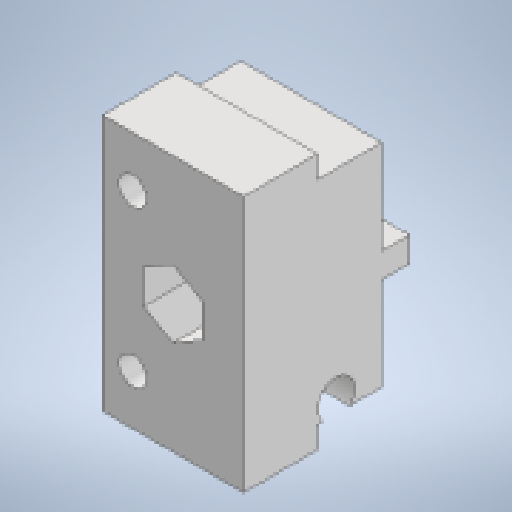
# Autodesk Inventor part: pokrywa silników
Saved by Autodesk Inventor 2023 (Build 270158000, 158)
## iProperties
Created: 2022-12-13
Part Number: pokrywa silników
Material: Generic
Document SubType Name: Modeling
Designer: komputer
Density: 1 g/cm^3
Appearance: Default
Author: komputer
Autodesk Inventor part; units mm, degrees
ref_plane "YZ Plane" through (0, 0, 0) normal (1, 0, 0) x (0, 1, 0)
ref_plane "XZ Plane" through (0, 0, 0) normal (0, 1, 0) x (-1, 0, 0)
ref_plane "XY Plane" through (0, 0, 0) normal (0, 0, 1) x (1, 0, 0)
sketch "Sketch1" plane through (0, 0, 0) normal (0, 0, 1) x (1, 0, 0)
  line L0 (-23.5108, -23.5) -> (0, -23.5) projected
  line L1 (0, -10) -> (0, -23.5) projected
  line L2 (0, -10) -> (-23, -10) projected
  line L3 (-23, 0) -> (-23, -10) projected
  line L4 (-23, 0) -> (7.65, 0) projected
  line L5 (7.65, 3) -> (-23, 3) projected
  line L6 (-23, 13) -> (-23, 3) projected
  line L7 (-23, 13) -> (0, 13) projected
  line L8 (0, 26.5) -> (0, 13) projected
  line L9 (-23.5108, 26.5) -> (0, 26.5) projected
  line L10 (0, 3.8) -> (14.8, 3.8) projected
  line L11 (0, 12.2) -> (14.8, 12.2) projected
  line L12 (14.8, -0.8) -> (0, -0.8) projected
  line L13 (14.8, -9.2) -> (0, -9.2) projected
  line L14 (0, 3.8) -> (0, -0.8)
  circle A0 centre (0, 1.5) radius 3.0601
  line L15 (0, -0.8) -> (3.8745, -4.6745)
  line L16 (0, -0.8) -> (5.4793, -0.8) construction
  line L17 (0, 3.8) -> (3.8745, 7.6745)
  line L18 (0, 3.8) -> (5.4793, 3.8) construction
  line L19 (0.6829, -1.4829) -> (11.7635, -1.4829)
  line L20 (11.7635, -1.4829) -> (11.7635, -8.6829)
  line L21 (11.7635, -8.6829) -> (0.6829, -8.6829)
  line L22 (0.6829, -8.6829) -> (0.6829, -1.4829)
  line L23 (0.6829, 4.4829) -> (11.1249, 4.4829)
  line L24 (11.1249, 4.4829) -> (11.1249, 11.6829)
  line L25 (11.1249, 11.6829) -> (0.6829, 11.6829)
  line L26 (0.6829, 11.6829) -> (0.6829, 4.4829)
  arc A1 (7.65, 3) -> (7.65, 0) centre (7.65, 1.5) ccw projected
  line L27 (-23.5108, 26.5) -> (-23.5108, -23.5) projected
  point P0 (0, 0)
  dimension "d0" = 45
  dimension "d1" = 45
  dimension "d2" = 7.2
  dimension "d3" = 7.2
  constraints: 26 end point, 4 horizontal, 4 parallel, 2 equal length, 2 perpendicular, 2 point on circle, 2 point on line, 1 centre point, 1 midpoint, 1 vertical
  measures "d0" angle of L15 L16
  measures "d1" angle of L18 L17
  measures "d2" distance of L19.end L20.end
  measures "d3" distance of L24.end L23.end
extrude "Extrusion1" add sketch "Sketch1" against normal blind 0.5 contours L26 L25 L24 L23 | L19 L20 L21 L22
sketch "Sketch2" plane through (0, 0, 0) normal (0, 0, 1) x (1, 0, 0)
  line L0 (-23.5108, -23.5) -> (0, -23.5) projected
  line L1 (0, -10) -> (0, -23.5) projected
  line L2 (0, -10) -> (-23, -10) projected
  line L3 (-23, 0) -> (-23, -10) projected
  line L4 (-23, 0) -> (7.65, 0) projected
  line L5 (7.65, 3) -> (-23, 3) projected
  line L6 (-23, 13) -> (-23, 3) projected
  line L7 (-23, 13) -> (0, 13) projected
  line L8 (0, 26.5) -> (0, 13) projected
  line L9 (-23.5108, 26.5) -> (0, 26.5) projected
  line L10 (0.6829, 11.6829) -> (0.6829, 4.4829) projected
  line L11 (0.6829, 4.4829) -> (11.1249, 4.4829) projected
  line L12 (11.1249, 4.4829) -> (11.1249, 11.6829) projected
  line L13 (0.6829, 11.6829) -> (0.6829, 4.4829) projected
  line L14 (0.6829, 4.4829) -> (11.1249, 4.4829) projected
  line L15 (11.1249, 4.4829) -> (11.1249, 11.6829) projected
  line L16 (11.1249, 11.6829) -> (0.6829, 11.6829) projected
  line L17 (11.7635, -8.6829) -> (11.7635, -1.4829) projected
  line L18 (11.7635, -1.4829) -> (0.6829, -1.4829) projected
  line L19 (0.6829, -1.4829) -> (0.6829, -8.6829) projected
  line L20 (0.6829, -8.6829) -> (11.7635, -8.6829) projected
  line L21 (-18.1, 3) -> (-18.1, 7) projected
  line L22 (-18.1, 9) -> (-18.1, 13) projected
  line L23 (-18.1, 0) -> (-18.1, -4) projected
  line L24 (-18.1, -10) -> (-18.1, -6) projected
  line L25 (0, 13) -> (0, 3)
  line L26 (0, 0) -> (0, -10)
  line L27 (-18.1, 13) -> (0, 13)
  line L28 (-18.1, 13) -> (-0.9053, 13)
  line L29 (-0.9053, 13) -> (-0.9053, 15)
  line L30 (-0.9053, 15) -> (-18.1, 15)
  line L31 (-18.1, 15) -> (-18.1, 13)
  line L32 (-18.1, -10) -> (-0.9053, -10)
  line L33 (-0.9053, -10) -> (-0.9053, -12)
  line L34 (-0.9053, -12) -> (-18.1, -12)
  line L35 (-18.1, -12) -> (-18.1, -10)
  line L36 (0, 13) -> (14.8, 13) projected
  line L37 (14.8, -10) -> (0, -10) projected
  line L38 (15.3, 13) -> (15.3, 12.2) projected
  line L39 (15.3, 0) -> (15.3, -0.8) projected
  line L40 (15.3, 13) -> (0, 13)
  line L41 (0, 13) -> (0, -10)
  line L42 (0, -10) -> (15.3, -10)
  line L43 (15.3, -10) -> (15.3, 13)
  arc A0 (7.65, 3) -> (7.65, 0) centre (7.65, 1.5) ccw projected
  line L44 (-23.5108, 26.5) -> (-23.5108, -23.5) projected
  point P0 (0, 3)
  dimension "d6" = 2
  dimension "d7" = 2
  constraints: 30 end point, 7 equal length, 5 perpendicular, 3 horizontal, 1 point on line
  measures "d6" distance of L29.end L28.end
  measures "d7" distance of L32.end L33.end
extrude "Extrusion2" add sketch "Sketch2" along normal blind 8 contours L26 L4 A0 L5 L25 L36 L40 L38 L43 L39 L42 L37 | L41 L5 A0 L4 | L16 L12 L11 L10 | L20 L19 L18 L17
sketch "Sketch3" plane through (0, 0, 8) normal (0, 0, 1) x (1, 0, 0)
  line L0 (15.3, -10) -> (15.3, 13) projected
  line L1 (15.3, 13) -> (0, 13) projected
  line L2 (0, 13) -> (0, -10) projected
  line L3 (0, -10) -> (15.3, -10) projected
  line L4 (-23.5108, -23.5) -> (0, -23.5) projected
  line L5 (0, -10) -> (0, -23.5) projected
  line L6 (0, -10) -> (-23, -10) projected
  line L7 (-23, 0) -> (-23, -10) projected
  line L8 (-23, 0) -> (7.65, 0) projected
  line L9 (7.65, 3) -> (-23, 3) projected
  line L10 (-23, 13) -> (-23, 3) projected
  line L11 (-23, 13) -> (0, 13) projected
  line L12 (0, 26.5) -> (0, 13) projected
  line L13 (-23.5108, 26.5) -> (0, 26.5) projected
  line L14 (9.34, 0) -> (13.34, 0) projected
  line L15 (9.34, 0.5) -> (13.34, 0.5) projected
  line L16 (9.34, 0) -> (13.34, 0)
  line L17 (13.34, 0) -> (13.34, 3)
  line L18 (13.34, 3) -> (9.34, 3)
  line L19 (9.34, 3) -> (9.34, 0)
  line L20 (0, -10) -> (15.3, -10) projected
  line L21 (0, -10) -> (15.3, -10)
  line L22 (7.65, -10) -> (7.65, 13)
  line L23 (15.3, 13) -> (0, 13) projected
  circle A0 centre (7.65, 1.5) radius 1.5
  circle A1 centre (7.65, 1.5) radius 4.5962
  line L24 (10.85, -0.3475) -> (10.85, 3.3475)
  line L25 (7.65, -2.195) -> (10.85, -0.3475)
  line L26 (4.45, -0.3475) -> (7.65, -2.195)
  line L27 (4.45, 3.3475) -> (4.45, -0.3475)
  line L28 (7.65, 5.195) -> (4.45, 3.3475)
  line L29 (10.85, 3.3475) -> (7.65, 5.195)
  arc A2 (7.65, 3) -> (7.65, 0) centre (7.65, 1.5) ccw projected
  line L30 (-23.5108, 26.5) -> (-23.5108, -23.5) projected
  point P0 (0, 0)
  point P1 (15.3, 0)
  point P2 (15.3, 3)
  dimension "d10" = 3
  constraints: 24 end point, 3 equal length, 3 midpoint, 2 centre point, 1 horizontal, 1 perpendicular, 1 point on line
  measures "d10" diameter of A0
extrude "Extrusion3" cut sketch "Sketch3" against normal blind 2 contours L26 L27 L8 L22 | L22 A0 L29 L24 L18 L19 L14 L25 | L22 L9 L27 L28 | L8 L27 L9 A0 | L14 L19 L15 L24 | L24 L15 L19 L18
sketch "Sketch4" plane through (7.65, 1.5, 8) normal (0, 0, 1) x (1, 0, 0)
  circle A0 centre (0, 0) radius 1.5 projected
  point P0 (-7.65, -1.5)
extrude "Extrusion4" cut sketch "Sketch4" against normal through all
sketch "Sketch5" plane through (0, 0, 0) normal (0, 0, -1) x (-1, 0, 0)
  line L0 (0, 3) -> (-14.8, 3) projected
  line L1 (-14.8, 0) -> (0, 0) projected
  line L2 (-14.8, 3) -> (-14.8, 2.8)
  line L3 (-15.3, -10) -> (-15.3, 13) projected
  line L4 (-14.8, 0) -> (-14.8, 0.2)
  line L5 (-14.8, 2.8) -> (-15.3, 2.8)
  line L6 (-15.3, 2.8) -> (-15.3, 0.1)
  line L7 (-15.3, 0.1) -> (-14.8, 0.1)
  line L8 (-14.8, 0.1) -> (-14.8, 2.8)
  line L9 (0, 13) -> (0, -10) projected
  line L10 (-15.3, 0.1) -> (0, 0.1)
  line L11 (0, 0.1) -> (0, 2.8)
  line L12 (0, 2.8) -> (-15.3, 2.8)
  line L13 (-15.3, 2.8) -> (-15.3, 0.1)
  circle A0 centre (-7.65, 1.5) radius 1.5 projected
  point P0 (-8.1885, 0.1)
  point P1 (-8.3983, 2.8)
  point P2 (-6.9017, 2.8)
  point P3 (-7.1115, 0.1)
  point P4 (0, 0.1)
  dimension "d15" = 0.2
  dimension "d16" = 0.2
  constraints: 20 end point, 5 parallel, 3 point on line, 2 horizontal, 2 perpendicular, 1 vertical
  measures "d15" distance of L0.end L2.end
  measures "d16" distance of L1.start L4.end
extrude "Extrusion5" add sketch "Sketch5" along normal blind 3 contours L9 L10 A0 L12 | A0 L10 L4 L8 L12
sketch "Sketch6" plane through (0, 0, 0) normal (0, 0, -1) x (-1, 0, 0)
  circle A0 centre (-7.65, 1.5) radius 2.5 projected
  line L0 (-15.3, 13) -> (-2.34, 13) projected
  line L1 (-15.3, -10) -> (-15.3, 13) projected
  line L2 (-2.34, -10) -> (-15.3, -10) projected
  line L3 (-14.8, 0.1) -> (-8.1885, 0.1) projected
  line L4 (-8.3983, 2.8) -> (-14.8, 2.8) projected
  line L5 (-14.8, 2.8) -> (-14.8, 0.1) projected
  line L6 (-15.3, -10) -> (-15.3, 13) projected
  line L7 (-14.8, 0.1) -> (-15.3, 0.1)
  line L8 (-15.3, 0.1) -> (-15.3, 2.8)
  line L9 (-15.3, 2.8) -> (-14.8, 2.8)
  line L10 (-14.8, 2.8) -> (-14.8, 0.1)
  line L11 (-2.34, -10) -> (-2.34, 13) projected
  point P0 (0, 0)
  constraints: 8 end point, 2 parallel, 1 horizontal, 1 perpendicular, 1 point on line
extrude "Extrusion6" add sketch "Sketch6" along normal blind 3 contours L5 L7 L1 L9
sketch "Sketch7" plane through (0, 0, 8) normal (0, 0, 1) x (1, 0, 0)
  line L0 (-17.2332, 12.8233) -> (-13.1798, 21.6639) projected
  line L1 (-17.2332, -10) -> (-17.2332, 12.8233) projected
  line L2 (-13.1798, -18.8406) -> (-17.2332, -10) projected
  line L3 (-13.1798, 21.6639) -> (15.3, 21.6639) projected
  line L4 (0, 13) -> (0, -10) projected
  circle A0 centre (7.65, 1.5) radius 1.5 projected
  circle A1 centre (7.65, 1.5) radius 7.65
  circle A2 centre (7.65, 1.5) radius 11.5
  line L5 (0, -10) -> (15.3, -10) projected
  line L6 (3.2816, -10) -> (3.2816, 13)
  line L7 (15.3, 13) -> (0, 13) projected
  line L8 (3.2816, -9.138) -> (3.2816, -4.7801)
  line L9 (3.2816, 7.7801) -> (3.2816, 12.138)
  circle A3 centre (3.2816, -6.9591) radius 1.5
  circle A4 centre (3.2816, 9.9591) radius 1.5
  line L10 (-13.1798, -18.8406) -> (15.3, -18.8406) projected
  line L11 (15.3, -18.8406) -> (15.3, 21.6639) projected
  circle A5 centre (3.2816, -6.9591) radius 1.5 projected
  circle A6 centre (3.2816, 9.9591) radius 1.5 projected
  point P0 (0, 0)
  point P1 (-1.7122, -18.8406)
  dimension "d21" = 3
  dimension "d22" = 3
  constraints: 6 end point, 6 point on line, 4 centre point, 4 point on circle, 2 coincident, 2 midpoint, 1 tangent
  measures "d21" diameter of A3
  measures "d22" diameter of A4
extrude "Extrusion7" cut sketch "Sketch7" against normal through all contours A4 L6 | L6 A4 | A3 L6 | L6 A3
sketch "Sketch8" plane through (0, 0, 8) normal (0, 0, 1) x (1, 0, 0)
  line L0 (0, -10) -> (15.3, -10) projected
  line L1 (15.3, -10) -> (15.3, 13) projected
  line L2 (0, 13) -> (0, -10) projected
  circle A0 centre (3.2816, -6.9591) radius 1.5 projected
  circle A1 centre (3.2816, 9.9591) radius 1.5 projected
  line L3 (15.3, 13) -> (0, 13) projected
  circle A2 centre (3.2816, -6.9591) radius 3.0409
  circle A3 centre (3.2816, 9.9591) radius 3.0409
  circle A4 centre (7.65, 1.5) radius 1.5 projected
  line L4 (10.85, 3.3475) -> (10.85, -0.3475) projected
  line L5 (10.85, 1.5) -> (15.3, 1.5)
  line L6 (15.3, -10) -> (10.85, -10)
  line L7 (10.85, -10) -> (10.85, 13)
  line L8 (10.85, 13) -> (15.3, 13)
  line L9 (15.3, 13) -> (15.3, -10)
  line L10 (10.85, -10) -> (15.3, -10)
  line L11 (15.3, -10) -> (15.3, -5.55)
  line L12 (15.3, -5.55) -> (10.85, -5.55)
  line L13 (10.85, -5.55) -> (10.85, -10)
  line L14 (15.3, 13) -> (10.85, 13)
  line L15 (10.85, 13) -> (10.85, 8.55)
  line L16 (10.85, 8.55) -> (15.3, 8.55)
  line L17 (15.3, 8.55) -> (15.3, 13)
  point P0 (0, 0)
  dimension "d25" = 4.45
  dimension "d26" = 4.45
  constraints: 26 end point, 6 parallel, 3 horizontal, 3 perpendicular, 3 point on line, 2 centre point, 2 coincident, 2 midpoint, 2 tangent
  measures "d25" distance of L11.end L10.end
  measures "d26" distance of L15.end L14.end
ref_plane "Work Plane1" through (-17.2332, -18.8406, 13) normal (0, 0, -1) x (0, 1, 0)
extrude "Extrusion8" add sketch "Sketch8" along normal up to surface (5 mm away) contours L7 L12 L1 L0 | A3 | A2 | L16 L7 L3 L1
fillet "Fillet1" radius 3 4 edges at (15.3, -10, 6.5) (15.3, 13, 6.5) (0, -10, 4) (0, 13, 4)
fillet "Fillet2" [suppressed]
sketch "Sketch9" plane through (10.85, 8.55, 13) normal (0, 0, 1) x (1, 0, 0)
  circle A0 centre (-7.5684, 1.4091) radius 1.5 projected
  circle A1 centre (-7.5684, 1.4091) radius 3.0409 projected
  line L0 (0, -8.8975) -> (-3.2, -10.745) projected
  line L1 (-3.2, -10.745) -> (-6.4, -8.8975) projected
  line L2 (-6.4, -8.8975) -> (-6.4, -5.2025) projected
  line L3 (-6.4, -5.2025) -> (-3.2, -3.355) projected
  line L4 (-3.2, -3.355) -> (0, -5.2025) projected
  line L5 (0, -5.2025) -> (0, -8.8975) projected
  arc A2 (-7.85, 4.45) -> (-10.85, 1.45) centre (-7.85, 1.45) ccw projected
  line L6 (-10.85, 1.45) -> (-10.85, -15.55) projected
  arc A3 (-10.85, -15.55) -> (-7.85, -18.55) centre (-7.85, -15.55) ccw projected
  line L7 (-7.85, -18.55) -> (-7.5684, -18.55) projected
  circle A4 centre (-7.5684, -15.5091) radius 3.0409 projected
  line L8 (-7.5684, -18.55) -> (0, -18.55) projected
  line L9 (0, -18.55) -> (0, -14.1) projected
  line L10 (0, -14.1) -> (4.45, -14.1) projected
  line L11 (4.45, -14.1) -> (4.45, 0) projected
  line L12 (4.45, 0) -> (0, 0) projected
  line L13 (0, 0) -> (0, 4.45) projected
  line L14 (0, 4.45) -> (-7.5684, 4.45) projected
  circle A5 centre (-7.5684, 1.4091) radius 3.0409 projected
  line L15 (-7.5684, 4.45) -> (-7.85, 4.45) projected
  arc A6 (4.45, 1.45) -> (1.45, 4.45) centre (1.45, 1.45) ccw projected
  line L16 (1.45, 4.45) -> (0, 4.45) projected
  line L17 (0, 4.45) -> (0, 0) projected
  line L18 (0, 0) -> (4.45, 0) projected
  line L19 (4.45, 0) -> (4.45, 1.45) projected
  arc A7 (1.45, -18.55) -> (4.45, -15.55) centre (1.45, -15.55) ccw projected
  line L20 (4.45, -15.55) -> (4.45, -14.1) projected
  line L21 (4.45, -14.1) -> (0, -14.1) projected
  line L22 (0, -14.1) -> (0, -18.55) projected
  line L23 (0, -18.55) -> (1.45, -18.55) projected
  point P0 (-10.85, -8.55)
  constraints: 2 vertical alignment
extrude "Extrusion9" cut sketch "Sketch9" against normal blind 10 contours L0 L1 L2 L3 L4 L5
sketch "Sketch10" plane through (10.85, 8.55, 13) normal (0, 0, 1) x (1, 0, 0)
  arc A0 (4.45, 1.45) -> (1.45, 4.45) centre (1.45, 1.45) ccw projected
  line L0 (0, -8.8975) -> (-3.2, -10.745) projected
  line L1 (-3.2, -10.745) -> (-6.4, -8.8975) projected
  line L2 (-6.4, -8.8975) -> (-6.4, -5.2025) projected
  line L3 (-6.4, -5.2025) -> (-3.2, -3.355) projected
  line L4 (-3.2, -3.355) -> (0, -5.2025) projected
  line L5 (0, -5.2025) -> (0, -8.8975) projected
  arc A1 (-7.85, 4.45) -> (-10.85, 1.45) centre (-7.85, 1.45) ccw projected
  line L6 (-10.85, 1.45) -> (-10.85, -15.55) projected
  arc A2 (-10.85, -15.55) -> (-7.85, -18.55) centre (-7.85, -15.55) ccw projected
  line L7 (-7.85, -18.55) -> (-7.5684, -18.55) projected
  circle A3 centre (-7.5684, -15.5091) radius 3.0409 projected
  line L8 (-7.5684, -18.55) -> (0, -18.55) projected
  line L9 (0, -18.55) -> (0, -14.1) projected
  line L10 (0, -14.1) -> (4.45, -14.1) projected
  line L11 (4.45, -14.1) -> (4.45, 0) projected
  line L12 (4.45, 0) -> (0, 0) projected
  line L13 (0, 0) -> (0, 4.45) projected
  line L14 (0, 4.45) -> (-7.5684, 4.45) projected
  circle A4 centre (-7.5684, 1.4091) radius 3.0409 projected
  line L15 (-7.5684, 4.45) -> (-7.85, 4.45) projected
  arc A5 (4.45, 1.45) -> (1.45, 4.45) centre (1.45, 1.45) ccw projected
  line L16 (1.45, 4.45) -> (0, 4.45) projected
  line L17 (0, 4.45) -> (0, 0) projected
  line L18 (0, 0) -> (4.45, 0) projected
  line L19 (4.45, 0) -> (4.45, 1.45) projected
  arc A6 (1.45, -18.55) -> (4.45, -15.55) centre (1.45, -15.55) ccw projected
  line L20 (4.45, -15.55) -> (4.45, -14.1) projected
  line L21 (4.45, -14.1) -> (0, -14.1) projected
  line L22 (0, -14.1) -> (0, -18.55) projected
  line L23 (0, -18.55) -> (1.45, -18.55) projected
  point P0 (-10.85, -8.55)
  point P1 (4.45, 1.45)
  point P2 (1.45, 4.45)
  constraints: 2 vertical alignment
extrude "Extrusion10" cut sketch "Sketch10" against normal blind 6 contours L19 L12 L13 L16 A0 | A4 | A3 | L11 L10 L9 L8 L7 A2 L6 A1 L15 L14 L13 L12 | L20 A6 L23 L9 L10 | L0 L1 L2 L3 L4 L5
sketch "Sketch11" plane through (10.85, 8.55, 7) normal (0, 0, 1) x (1, 0, 0)
  circle A0 centre (-7.5684, 1.4091) radius 1.5 projected
  circle A1 centre (-7.5684, -15.5091) radius 1.5 projected
  line L0 (-3.2, -10.745) -> (0, -8.8975) projected
  line L1 (-6.4, -8.8975) -> (-3.2, -10.745) projected
  line L2 (-6.4, -5.2025) -> (-6.4, -8.8975) projected
  line L3 (-3.2, -3.355) -> (-6.4, -5.2025) projected
  line L4 (0, -5.2025) -> (-3.2, -3.355) projected
  line L5 (0, -8.8975) -> (0, -5.2025) projected
  line L6 (1.45, -18.55) -> (-7.85, -18.55) projected
  arc A2 (1.45, -18.55) -> (4.45, -15.55) centre (1.45, -15.55) ccw projected
  line L7 (4.45, 1.45) -> (4.45, -15.55) projected
  arc A3 (4.45, 1.45) -> (1.45, 4.45) centre (1.45, 1.45) ccw projected
  line L8 (-7.85, 4.45) -> (1.45, 4.45) projected
  arc A4 (-7.85, 4.45) -> (-10.85, 1.45) centre (-7.85, 1.45) ccw projected
  line L9 (-10.85, -15.55) -> (-10.85, 1.45) projected
  arc A5 (-10.85, -15.55) -> (-7.85, -18.55) centre (-7.85, -15.55) ccw projected
  line L10 (-10.85, 4.45) -> (4.45, 4.45)
  line L11 (4.45, 4.45) -> (4.45, -18.55)
  line L12 (4.45, -18.55) -> (-10.85, -18.55)
  line L13 (-10.85, -18.55) -> (-10.85, 4.45)
  point P0 (-10.85, -8.55)
  point P1 (1.45, 4.45)
  constraints: 8 end point, 2 parallel, 1 horizontal, 1 perpendicular
extrude "Extrusion11" add sketch "Sketch11" against normal up to surface (7 mm away) contours A2 L11 L12 | L12 L13 A5 | A3 L10 L11 | L13 L10 A4
sketch "Sketch12" plane through (0, 2.8, 0) normal (-1, 0, 0) x (0, 0, 1)
  line L0 (6.5, 12.6142) -> (14.5, 12.6142) projected
  line L1 (7, -12.8) -> (7, 10.2) projected
  line L2 (7, 10.2) -> (0, 10.2) projected
  line L3 (0, 10.2) -> (0, 0) projected
  line L4 (0, 0) -> (-3, 0) projected
  line L5 (-3, -2.7) -> (-3, 0) projected
  line L6 (0, -2.7) -> (-3, -2.7) projected
  line L7 (0, -12.8) -> (0, -2.7) projected
  line L8 (7, -12.8) -> (0, -12.8) projected
  line L9 (7, -12.8) -> (7, 10.2) projected
  line L10 (7, -1.3) -> (-6.3728, -1.3)
  line L11 (12, 18.5) -> (0, 18.5) projected
  line L12 (0, 18.5) -> (0, -21.5) projected
  line L13 (12, -21.5) -> (0, -21.5) projected
  line L14 (12, 18.5) -> (12, -21.5) projected
  line L15 (12, 12.2747) -> (15, 12.2747)
  line L16 (7, 10.2) -> (15, 10.2)
  line L17 (15, 10.2) -> (15, 12.6142)
  line L18 (15, 12.6142) -> (7, 12.6142)
  line L19 (7, 12.6142) -> (7, 10.2)
  line L20 (7, -1.3) -> (15, -1.3)
  line L21 (15, -1.3) -> (15, 12.6142)
  line L22 (15, 12.6142) -> (7, 12.6142)
  line L23 (7, 12.6142) -> (7, -1.3)
  line L24 (6.5, -15.2142) -> (14.5, -15.2142)
  line L25 (15, -15.2142) -> (7, -15.2142)
  line L26 (15, -1.3) -> (15, -15.2142)
  line L27 (7, -15.2142) -> (7, -1.3)
  point P0 (0, -2.8)
  dimension "d37" = 3
  constraints: 28 end point, 5 symmetric about line, 4 parallel, 3 horizontal, 3 perpendicular, 1 midpoint, 1 point on line
  measures "d37" distance of L15.start L15.end
extrude "Extrusion12" add sketch "Sketch12" against normal up to surface (15.3 mm away) contours L0 L14 L16 L19 | L0 L18 L17 L15 L14 | L16 L14 L20 L1 | L15 L17 L16 L14 | L20 L14 L24 L27 L1 | L16 L21 L20 L14 | L20 L26 L25 L24 L14
sketch "Sketch13" plane through (0, -12.4142, 15) normal (0, 0, 1) x (1, 0, 0)
  line L0 (10.85, 15.7617) -> (10.85, 12.0667) projected
  line L1 (10.85, 15.7617) -> (7.65, 17.6093) projected
  line L2 (7.65, 17.6093) -> (4.45, 15.7617) projected
  line L3 (4.45, 15.7617) -> (4.45, 12.0667) projected
  line L4 (7.65, 10.2192) -> (4.45, 12.0667) projected
  line L5 (7.65, 10.2192) -> (10.85, 12.0667) projected
  circle A0 centre (7.65, 13.9142) radius 1.5 projected
  circle A1 centre (3.2816, 22.3733) radius 1.5 projected
  line L6 (0, 25.4142) -> (0, 15.2142) projected
  line L7 (0, 12.5142) -> (0, 15.2142) projected
  line L8 (0, 2.4142) -> (0, 12.5142) projected
  line L9 (0, 2.4142) -> (0, 0) projected
  line L10 (0, 0) -> (0, 27.8284) projected
  line L11 (0, 27.8284) -> (0, 25.4142) projected
  circle A2 centre (3.2816, 5.4552) radius 1.5 projected
  point P0 (0, 12.4142)
extrude "Extrusion13" cut sketch "Sketch13" against normal up to surface (15 mm away) contours L0 L5 L4 L3 L2 L1 | A0 | A1 | A2
sketch "Sketch14" plane through (8.1885, 0.1, 0) normal (0, 0, 1) x (1, 0, 0)
  circle A0 centre (-4.9069, 9.8591) radius 1.5 projected
  line L0 (-3.7385, 3.2475) -> (-0.5385, 5.095) projected
  line L1 (-0.5385, 5.095) -> (2.6615, 3.2475) projected
  line L2 (2.6615, 3.2475) -> (2.6615, -0.4475) projected
  line L3 (2.6615, -0.4475) -> (-0.5385, -2.295) projected
  line L4 (-0.5385, -2.295) -> (-3.7385, -0.4475) projected
  line L5 (-3.7385, -0.4475) -> (-3.7385, 3.2475) projected
  circle A1 centre (-4.9069, -7.0591) radius 1.5 projected
  line L6 (7.1115, -12.5142) -> (7.1115, 15.3142) projected
  line L7 (-8.1885, 15.3142) -> (7.1115, 15.3142) projected
  line L8 (-8.1885, -12.5142) -> (-8.1885, 15.3142) projected
  line L9 (-8.1885, -12.5142) -> (7.1115, -12.5142) projected
  arc A2 (0, 0) -> (0.2098, 2.7) centre (-0.5385, 1.4) ccw projected
  arc A3 (-1.2868, 2.7) -> (-1.077, 0) centre (-0.5385, 1.4) ccw projected
  circle A4 centre (-0.5385, 1.4) radius 1.5
  point P0 (-8.1885, -0.1)
  point P1 (0, 0)
  point P2 (-1.077, 0)
  point P3 (0.2098, 2.7)
  constraints: 1 centre point, 1 coincident
extrude "Extrusion14" add sketch "Sketch14" along normal blind 3 contours L0 L1 L2 L3 L4 L5
sketch "Szkic15" plane through (0, 2.8, 0) normal (-1, 0, 0) x (0, 0, 1)
  line L0 (7, 10.2) -> (0, 10.2) projected
  line L1 (0, 10.2) -> (0, 0) projected
  line L2 (0, 0) -> (-3, 0) projected
  line L3 (-3, -2.7) -> (-3, 0) projected
  line L4 (0, -2.7) -> (-3, -2.7) projected
  line L5 (0, -12.8) -> (0, -2.7) projected
  line L6 (7, -12.8) -> (0, -12.8) projected
  line L7 (7, -12.8) -> (7, -15.2142) projected
  line L8 (7, -15.2142) -> (15, -15.2142) projected
  line L9 (15, -15.2142) -> (15, 12.6142) projected
  line L10 (15, 12.6142) -> (7, 12.6142) projected
  line L11 (7, 12.6142) -> (7, 10.2) projected
  circle A0 centre (4.9651, -11.4206) radius 2
  point P0 (0, -2.8)
  dimension "d44" = 4
  constraints: 1 centre point
  measures "d44" diameter of A0
extrude "Wyciągnięcie proste15" cut sketch "Szkic15" against normal through all contours A0 L6 | L6 A0
sketch "Szkic16" plane through (0, -12.4142, 15) normal (0, 0, 1) x (1, 0, 0)
  circle A0 centre (3.2816, 22.3733) radius 1.5 projected
  line L0 (4.45, 15.7617) -> (7.65, 17.6093) projected
  line L1 (7.65, 17.6093) -> (10.85, 15.7617) projected
  line L2 (10.85, 15.7617) -> (10.85, 12.0667) projected
  line L3 (10.85, 12.0667) -> (7.65, 10.2192) projected
  line L4 (7.65, 10.2192) -> (4.45, 12.0667) projected
  line L5 (4.45, 12.0667) -> (4.45, 15.7617) projected
  circle A1 centre (3.2816, 5.4552) radius 1.5 projected
  line L6 (15.3, 0) -> (15.3, 27.8284) projected
  line L7 (0, 27.8284) -> (15.3, 27.8284) projected
  line L8 (0, 0) -> (0, 27.8284) projected
  line L9 (0, 0) -> (15.3, 0) projected
  line L10 (3.2816, 22.3733) -> (7.2816, 22.3733)
  line L11 (3.2816, 5.4552) -> (7.2816, 5.4552)
  circle A2 centre (7.2816, 22.3733) radius 1.5
  circle A3 centre (7.2816, 5.4552) radius 1.5
  point P0 (0, 12.4142)
  dimension "d47" = 4
  dimension "d48" = 4
  constraints: 4 end point, 2 centre point, 2 coincident, 2 horizontal
  measures "d47" distance of L10.start L10.end
  measures "d48" distance of L11.start L11.end
extrude "Wyciągnięcie proste16" cut sketch "Szkic16" against normal through all contours A2 | A3
fillet "Zaokrąglenie3" radius 4 4 edges at (7.65, 13, 7) (7.65, 15.4142, 7) (7.65, -10, 7) (7.65, -12.4142, 7)
fillet "Zaokrąglenie5" radius 0.5 28 edges at (0, 15.4142, 12.8361) (0, 13.3141, 6.499) (0, 13, 2.4726) (0, 15.1001, 9.1185) (0, -12.0344, 8.971) (0, -12.4142, 12.8361) (0, -10.4268, 7.0496) (0, -10, 1.7585) (0, -6.7637, 4.2223) (0, -9.3182, 6.8395) (0, -9.9645, 6.4464) (15.3, -12.4142, 12.8361) (15.3, -10.4268, 7.0496) (15.3, -12.0344, 8.971) (15.3, -6.7637, 4.2223) (15.3, -9.3182, 6.8395) (15.3, -9.9645, 6.4464) (15.3, -10, 1.7585) (15.3, 13.3141, 6.499) (15.3, 15.1001, 9.1185) (15.3, 15.4142, 12.8361) (15.3, 13, 2.4726) (15.3, -4.95, 0) (15.3, 7.9, 0) (0, 7.9, 0) (0, -4.95, 0) (7.65, -10, 0) (7.65, 13, 0)
sketch "Szkic17" plane through (0, -11.9142, 15) normal (0, 0, 1) x (1, 0, 0)
  circle A0 centre (3.2816, 4.9552) radius 1.5 projected
  line L0 (4.45, 15.2617) -> (7.65, 17.1093) projected
  line L1 (7.65, 17.1093) -> (10.85, 15.2617) projected
  line L2 (10.85, 15.2617) -> (10.85, 11.5667) projected
  line L3 (10.85, 11.5667) -> (7.65, 9.7192) projected
  line L4 (7.65, 9.7192) -> (4.45, 11.5667) projected
  line L5 (4.45, 11.5667) -> (4.45, 15.2617) projected
  circle A1 centre (3.2816, 21.8733) radius 1.5 projected
  circle A2 centre (7.2816, 21.8733) radius 1.5 projected
  circle A3 centre (7.2816, 4.9552) radius 1.5 projected
  arc A4 (0, 0) -> (0.5, -0.5) centre (0.5, 0) ccw projected
  line L6 (0.5, -0.5) -> (14.8, -0.5) projected
  arc A5 (14.8, -0.5) -> (15.3, 0) centre (14.8, 0) ccw projected
  line L7 (15.3, 0) -> (15.3, 26.8284) projected
  arc A6 (15.3, 26.8284) -> (14.8, 27.3284) centre (14.8, 26.8284) ccw projected
  line L8 (0.5, 27.3284) -> (14.8, 27.3284) projected
  arc A7 (0.5, 27.3284) -> (0, 26.8284) centre (0.5, 26.8284) ccw projected
  line L9 (0, 0) -> (0, 26.8284) projected
  point P0 (0, 11.9142)
extrude "Wyciągnięcie proste17" add sketch "Szkic17" along normal blind 2
sketch "Szkic18" plane through (0, -11.9142, 17) normal (0, 0, 1) x (1, 0, 0)
  line L0 (0, 26.8284) -> (0, 0) projected
  arc A0 (0, 0) -> (0.5, -0.5) centre (0.5, 0) ccw projected
  line L1 (0.5, -0.5) -> (14.8, -0.5) projected
  arc A1 (14.8, -0.5) -> (15.3, 0) centre (14.8, 0) ccw projected
  line L2 (15.3, 0) -> (15.3, 26.8284) projected
  arc A2 (15.3, 26.8284) -> (14.8, 27.3284) centre (14.8, 26.8284) ccw projected
  line L3 (14.8, 27.3284) -> (0.5, 27.3284) projected
  arc A3 (0.5, 27.3284) -> (0, 26.8284) centre (0.5, 26.8284) ccw projected
  circle A4 centre (3.2816, 4.9552) radius 1.5 projected
  circle A5 centre (3.2816, 21.8733) radius 1.5 projected
  circle A6 centre (7.2816, 21.8733) radius 1.5 projected
  circle A7 centre (7.2816, 4.9552) radius 1.5 projected
  line L4 (4.45, 15.2617) -> (7.65, 17.1093) projected
  line L5 (7.65, 17.1093) -> (10.85, 15.2617) projected
  line L6 (10.85, 15.2617) -> (10.85, 11.5667) projected
  line L7 (10.85, 11.5667) -> (7.65, 9.7192) projected
  line L8 (7.65, 9.7192) -> (4.45, 11.5667) projected
  line L9 (4.45, 11.5667) -> (4.45, 15.2617) projected
  line L10 (0, 2.4142) -> (0, 12.0142) projected
  line L11 (15.3, 15.2617) -> (0, 15.2617)
  line L12 (0, 15.2617) -> (0, 11.5667)
  line L13 (0, 11.5667) -> (15.3, 11.5667)
  line L14 (15.3, 11.5667) -> (15.3, 15.2617)
  line L15 (0, 15.2617) -> (15.3, 15.2617)
  line L16 (15.3, 15.2617) -> (15.3, 18.5718)
  line L17 (15.3, 18.5718) -> (0, 18.5718)
  line L18 (0, 18.5718) -> (0, 15.2617)
  line L19 (15.3, 13.4142) -> (18.3704, 13.4142)
  line L20 (15.3, 8.2567) -> (0, 8.2567)
  point P0 (0, 11.9142)
  point P1 (0, 18.5718)
  point P2 (0, 8.2567)
  point P3 (15.3, 8.2567)
  constraints: 20 end point, 4 parallel, 3 horizontal, 3 point on line, 2 perpendicular, 2 symmetric about line, 1 midpoint
extrude "Wyciągnięcie proste18" cut sketch "Szkic18" against normal blind 10 contours L17 L2 L11 L5 L4 L0 | L11 L9 L13 L0 | L2 L13 L6 L11 | L13 L8 L7 L2 L20 L0
fillet "Zaokrąglenie6" radius 2 2 edges at (7.65, 6.6575, 7) (7.65, -3.6575, 7)
fillet "Zaokrąglenie7" radius 0.5 22 edges at (7.65, 6.6575, 17) (0, 6.0718, 7.5858) (0, 1.5, 7) (0, -3.0718, 7.5858) (0, -3.6575, 13) (0, 6.6575, 13) (7.65, -3.6575, 17) (15.3, 1.5, 7) (15.3, 6.0718, 7.5858) (15.3, 6.6575, 13) (15.3, -3.6575, 13) (15.3, -3.0718, 7.5858) (15.1536, 15.2678, 17) (7.65, 15.4142, 17) (0.1464, 15.2678, 17) (0, 10.7859, 17) (15.3, 10.7859, 17) (15.1536, -12.2678, 17) (7.65, -12.4142, 17) (0.1464, -12.2678, 17) (0, -7.7859, 17) (15.3, -7.7859, 17)
sketch "Szkic19" plane through (8.1885, 0.1, 3) normal (0, 0, 1) x (1, 0, 0)
  circle A0 centre (-0.5385, 1.4) radius 1.5 projected
  circle A1 centre (-0.5385, 1.4) radius 1.75
  point P0 (-8.1885, -0.1)
  dimension "d60" = 3.5
  constraints: 1 centre point, 1 coincident
  measures "d60" diameter of A1
extrude "Wyciągnięcie proste19" cut sketch "Szkic19" against normal through all contours A0 | A1
fillet "Zaokrąglenie8" radius 0.1 4 edges at (0, 0.1, -1.5) (0, 2.8, -1.25) (15.3, 0.1, -1.25) (15.3, 2.8, -1.25)
fillet "Zaokrąglenie9" radius 0.3 10 edges at (15.2707, 0.1293, -3) (15.3, 1.45, -3) (15.2707, 2.7707, -3) (12.0108, 2.8, -3) (11.95, 0.1, -3) (0.0293, 0.1293, -3) (0, 1.45, -3) (0.0293, 2.7707, -3) (3.2892, 2.8, -3) (3.35, 0.1, -3)
body "Solid1"
